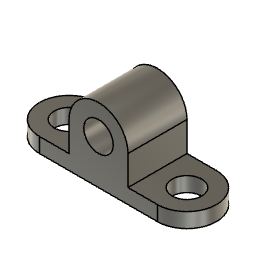
A4 (Autodesk Fusion 360 design; units mm, degrees)
Autodesk Fusion 360 part; units mm, degrees
sketch "Sketch1" plane through (0, 0, 0) normal (0, 0, 1) x (1, 0, 0)
  line L0 (40, 20) -> (-40, 20)
  line L1 (-40, -20) -> (40, -20)
  circle A0 centre (-40, 0) radius 10
  circle A1 centre (40, 0) radius 10
  line L2 (20, 0) -> (40, 0) construction
  arc A2 (40, -20) -> (40, 20) centre (40, 0) ccw
  arc A3 (-40, 20) -> (-40, -20) centre (-40, 0) ccw
  dimension "d1" = 80
  dimension "d2" = 40
  constraint horizontal L0
  constraint parallel L0 L1
  constraint coincident A1.centre L2.end
  measures "d1" distance of L1.start L1.end
  measures "d2" distance of L0.end L1.start
extrude "Extrude1" add sketch "Sketch1" along normal blind 10
sketch "Sketch2" plane through (0, -20, 0) normal (0, -1, 0) x (1, 0, 0)
  line L0 (-40, 0) -> (40, 0)
  line L1 (40, 0) -> (40, 10)
  line L2 (40, 10) -> (-40, 10)
  line L3 (-40, 10) -> (-40, 0)
  line L4 (-20, 0) -> (20, 0)
  line L5 (20, 0) -> (20, 30)
  line L6 (-20, 30) -> (-20, 0)
  circle A0 centre (0, 30) radius 10
  arc A1 (20, 30) -> (-20, 30) centre (0, 30) ccw
  dimension "d11" = 40
  dimension "d12" = 30
  dimension "d13" = 20
  dimension "d14" = 20
  dimension "d15" = 40
  constraint horizontal L4
  constraint vertical L5
  constraint vertical L6
  constraint coincident L0 L4.start
  constraint concentric A0 A1
  measures "d11" distance of L4.start L4.end
  measures "d12" distance of L4.start L6.start
  measures "d13" distance of L1 L5
  measures "d14" diameter of A0
  measures "d15" diameter of A1
extrude "Extrude2" add sketch "Sketch2" against normal blind 40 contours L2 L5 L6 A1
